Autodesk Fusion 360 part; units mm, degrees
(part 2 of 2)
  spline S18 degree 5 poles (-6.5449, 6.7429) (-6.5503, 6.7485) (-6.5613, 6.7594) (-6.5783, 6.7752) (-6.602, 6.7952) (-6.633, 6.8186) (-6.6649, 6.8409) (-6.6975, 6.8626) (-6.7305, 6.8839) (-6.7637, 6.905) (-6.7971, 6.9257) (-6.8309, 6.9462) (-6.8651, 6.9661) (-6.8998, 6.9854) (-6.9349, 7.0042) (-6.9705, 7.0225) (-7.0064, 7.0403) (-7.0427, 7.0577) (-7.0792, 7.0748) (-7.116, 7.0916) (-7.153, 7.108) (-7.1903, 7.1241) (-7.2279, 7.1398) (-7.2657, 7.1551) (-7.3038, 7.1701) (-7.3422, 7.1847) (-7.3809, 7.1989) (-7.4197, 7.2128) (-7.4588, 7.2264) (-7.4982, 7.2396) (-7.5377, 7.2526) (-7.5775, 7.2652) (-7.6174, 7.2774) (-7.6576, 7.2894) (-7.698, 7.301) (-7.7386, 7.3123) (-7.7793, 7.3233) (-7.8203, 7.334) (-7.8615, 7.3444) (-7.9028, 7.3544) (-7.9443, 7.3642) (-7.986, 7.3737) (-8.0279, 7.3828) (-8.07, 7.3916) (-8.1122, 7.4002) (-8.1545, 7.4084) (-8.1971, 7.4164) (-8.2398, 7.424) (-8.2826, 7.4313) (-8.3256, 7.4384) (-8.3688, 7.4451) (-8.4121, 7.4516) (-8.4555, 7.4577) (-8.4991, 7.4636) (-8.5429, 7.4692) (-8.5867, 7.4745) (-8.6307, 7.4795) (-8.6749, 7.4842) (-8.7191, 7.4886) (-8.7635, 7.4927) (-8.808, 7.4965) (-8.8527, 7.5001) (-8.8974, 7.5034) (-8.9423, 7.5063) (-8.9873, 7.509) (-9.0324, 7.5114) (-9.0777, 7.5136) (-9.123, 7.5154) (-9.1684, 7.5169) (-9.214, 7.5182) (-9.2596, 7.5192) (-9.2962, 7.5198) (-9.3237, 7.52) (-9.3421, 7.5202) (-9.3513, 7.5202) knots 0 0 0 0 0 0 0.01428571 0.02857143 0.04285714 0.05714286 0.07142857 0.08571429 0.1 0.11428571 0.12857143 0.14285714 0.15714286 0.17142857 0.18571429 0.2 0.21428571 0.22857143 0.24285714 0.25714286 0.27142857 0.28571429 0.3 0.31428571 0.32857143 0.34285714 0.35714286 0.37142857 0.38571429 0.4 0.41428571 0.42857143 0.44285714 0.45714286 0.47142857 0.48571429 0.5 0.51428571 0.52857143 0.54285714 0.55714286 0.57142857 0.58571429 0.6 0.61428571 0.62857143 0.64285714 0.65714286 0.67142857 0.68571429 0.7 0.71428571 0.72857143 0.74285714 0.75714286 0.77142857 0.78571429 0.8 0.81428571 0.82857143 0.84285714 0.85714286 0.87142857 0.88571429 0.9 0.91428571 0.92857143 0.94285714 0.95714286 0.97142857 0.98571429 1 1 1 1 1 1
  arc A38 (-9.3513, 7.5202) -> (-10.0419, 6.5697) centre (0, 0) ccw
  spline S19 degree 5 poles (-10.0419, 6.5697) (-10.039, 6.561) (-10.0332, 6.5436) (-10.0244, 6.5175) (-10.0126, 6.4829) (-9.9975, 6.4398) (-9.9822, 6.3968) (-9.9667, 6.3541) (-9.951, 6.3115) (-9.935, 6.2692) (-9.9187, 6.227) (-9.9023, 6.1851) (-9.8856, 6.1433) (-9.8686, 6.1017) (-9.8515, 6.0604) (-9.8341, 6.0192) (-9.8164, 5.9783) (-9.7986, 5.9376) (-9.7804, 5.897) (-9.7621, 5.8567) (-9.7435, 5.8166) (-9.7247, 5.7768) (-9.7056, 5.7371) (-9.6864, 5.6977) (-9.6668, 5.6585) (-9.6471, 5.6196) (-9.6271, 5.5808) (-9.6069, 5.5424) (-9.5864, 5.5041) (-9.5657, 5.4661) (-9.5448, 5.4283) (-9.5236, 5.3908) (-9.5022, 5.3536) (-9.4806, 5.3166) (-9.4587, 5.2799) (-9.4366, 5.2434) (-9.4142, 5.2072) (-9.3917, 5.1712) (-9.3688, 5.1356) (-9.3458, 5.1002) (-9.3225, 5.0651) (-9.299, 5.0303) (-9.2752, 4.9957) (-9.2511, 4.9615) (-9.2269, 4.9276) (-9.2024, 4.894) (-9.1776, 4.8607) (-9.1526, 4.8277) (-9.1274, 4.795) (-9.1019, 4.7627) (-9.0762, 4.7307) (-9.0502, 4.699) (-9.0239, 4.6678) (-8.9973, 4.6369) (-8.9705, 4.6064) (-8.9435, 4.5763) (-8.9162, 4.5465) (-8.8886, 4.517) (-8.8608, 4.4879) (-8.8328, 4.4593) (-8.8044, 4.4311) (-8.7757, 4.4035) (-8.7466, 4.3765) (-8.7171, 4.3501) (-8.6872, 4.3243) (-8.6571, 4.2989) (-8.6268, 4.2738) (-8.5964, 4.2491) (-8.5657, 4.2248) (-8.5346, 4.2013) (-8.5027, 4.179) (-8.4764, 4.1627) (-8.4561, 4.1514) (-8.4423, 4.1443) (-8.4354, 4.1409) knots -1 -1 -1 -1 -1 -1 -0.98571429 -0.97142857 -0.95714286 -0.94285714 -0.92857143 -0.91428571 -0.9 -0.88571429 -0.87142857 -0.85714286 -0.84285714 -0.82857143 -0.81428571 -0.8 -0.78571429 -0.77142857 -0.75714286 -0.74285714 -0.72857143 -0.71428571 -0.7 -0.68571429 -0.67142857 -0.65714286 -0.64285714 -0.62857143 -0.61428571 -0.6 -0.58571429 -0.57142857 -0.55714286 -0.54285714 -0.52857143 -0.51428571 -0.5 -0.48571429 -0.47142857 -0.45714286 -0.44285714 -0.42857143 -0.41428571 -0.4 -0.38571429 -0.37142857 -0.35714286 -0.34285714 -0.32857143 -0.31428571 -0.3 -0.28571429 -0.27142857 -0.25714286 -0.24285714 -0.22857143 -0.21428571 -0.2 -0.18571429 -0.17142857 -0.15714286 -0.14285714 -0.12857143 -0.11428571 -0.1 -0.08571429 -0.07142857 -0.05714286 -0.04285714 -0.02857143 -0.01428571 0 0 0 0 0 0
  line L19 (-8.4354, 4.1409) -> (-7.6212, 3.7403)
  arc A39 (-7.1196, 2.5104) -> (-7.6212, 3.7403) centre (-8.0626, 2.843) ccw
  circle A40 centre (0, 0) radius 17.5
  dimension "d9" = 35
  constraint concentric A0 A40
  measures "d9" diameter of A40
extrude "Extrude3" add sketch "Sketch1 (2)" along normal blind 7 contours A0 A1 L0 S0 A2 S1 L1 A3 A4 A5 L2 S2 A6 S3 L3 A7 A8 A9 L4 S4 A10 S5 L5 A11 A12 A13 L6 S6 A14 S7 L7 A15 A16 A17 L8 S8 A18 S9 L9 A19 A20 A21 L10 S10 A22 S11 L11 A23 A24 A25 L12 S12 A26 S13 L13 A27 A28 A29 L14 S14 A30 S15 L15 A31 A32 A33 L16 S16 A34 S17 L17 A35 A36 A37 L18 S18 A38 S19 L19 A39 | A40 in component "Spur Gear (10 teeth)"
sketch "Sketch2 (2)" plane through (0, 0, 38) normal (0, 0, 1) x (-1, 0, 0)
  line L0 (-3.5, -6.0622) -> (3.5, -6.0622)
  line L1 (3.5, -6.0622) -> (7, 0)
  line L2 (7, 0) -> (3.5, 6.0622)
  line L3 (3.5, 6.0622) -> (-3.5, 6.0622)
  line L4 (-3.5, 6.0622) -> (-7, 0)
  line L5 (-7, 0) -> (-3.5, -6.0622)
  circle A0 centre (0, 0) radius 5.75
extrude "Extrude4" cut sketch "Sketch2 (2)" against normal blind 31 contours L0 L1 L2 L3 L4 L5 | A0 in component "Spur Gear (10 teeth)"
component "Spur Gear (10 teeth)" placed x (1, 0, 0) y (0, 1, 0) z (0, 0, 1) at (0, 0, 0)
